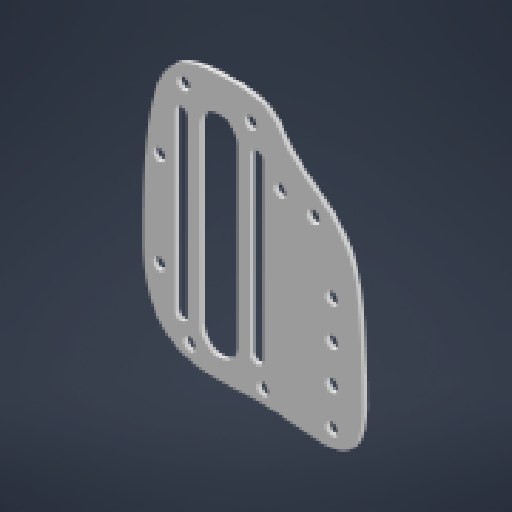
# Autodesk Inventor part: first-stage
Saved by Autodesk Inventor 2023.2 (Build 272271000, 271)
## iProperties
Created: 2023-03-31
Part Number: first-stage
Material: Generic
Document SubType Name: Modeling
Designer: eduar
Density: 1 g/cm^3
Appearance: Default
Author: eduar
Autodesk Inventor part; units mm, degrees
ref_plane "YZ Plane" through (0, 0, 0) normal (1, 0, 0) x (0, 1, 0)
ref_plane "XZ Plane" through (0, 0, 0) normal (0, 1, 0) x (-1, 0, 0)
ref_plane "XY Plane" through (0, 0, 0) normal (0, 0, 1) x (1, 0, 0)
sketch "Sketch1" plane through (0, 0, 0) normal (0, 0, 1) x (1, 0, 0)
  circle A0 centre (0, 139.7) radius 2.0955
  circle A1 centre (0, 127) radius 2.0955
  line L0 (-63.6282, 137.6045) -> (-63.6282, 111.7262) construction
  line L1 (-63.6282, 111.7262) -> (-38.1, 106.8497) construction
  line L2 (-38.1, 106.8497) -> (-23.3045, 114.3) construction
  line L3 (-23.3045, 114.3) -> (10.2927, 101.7972) construction
  line L4 (10.2927, 101.7972) -> (10.9951, 128.4781) construction
  line L5 (10.9951, 128.4781) -> (9.5904, 142.0848) construction
  line L6 (9.5904, 142.0848) -> (9.5904, 176.1435) construction
  line L7 (9.5904, 176.1435) -> (-18.114, 184.6297) construction
  line L8 (-18.114, 184.6297) -> (-19.6095, 190.621) construction
  line L9 (-19.6095, 190.621) -> (-43.1752, 188.9709) construction
  line L10 (-43.1752, 188.9709) -> (-63.6282, 188.9709) construction
  line L11 (-63.6282, 188.9709) -> (-63.6282, 149.1308) construction
  line L12 (-63.6282, 149.1308) -> (-63.6282, 137.6045) construction
  spline S0 degree 4 poles (-63.6282, 137.6045) (-63.6282, 111.7262) (-38.1, 106.8497) (-23.3045, 114.3) (10.2927, 101.7972) (10.9951, 128.4781) (9.5904, 142.0848) (9.5904, 176.1435) (-18.114, 184.6297) (-19.6095, 190.621) (-43.1752, 188.9709) (-63.6282, 188.9709) (-63.6282, 149.1308) (-63.6282, 137.6045) knots 0 0 0 0 0 1 2 3 4 5 6 7 8 9 10 10 10 10 10
  circle A2 centre (0, 114.3) radius 2.0955
  circle A3 centre (0, 152.4) radius 2.0955
  arc A4 (-31.75, 180.975) -> (-44.45, 180.975) centre (-38.1, 180.975) ccw
  line L13 (-44.45, 180.975) -> (-44.45, 122.555)
  line L14 (-31.75, 180.975) -> (-31.75, 122.555)
  arc A5 (-48.7045, 180.975) -> (-52.8955, 180.975) centre (-50.8, 180.975) ccw
  line L15 (-52.8955, 180.975) -> (-48.7045, 180.975) construction
  line L16 (-44.45, 180.975) -> (-31.75, 180.975) construction
  arc A6 (-23.3045, 180.975) -> (-27.4955, 180.975) centre (-25.4, 180.975) ccw
  line L17 (-23.3045, 180.975) -> (-27.4955, 180.975) construction
  line L18 (-23.3045, 180.975) -> (-23.3045, 122.555)
  line L19 (-27.4955, 180.975) -> (-27.4955, 122.555)
  line L20 (-48.7045, 180.975) -> (-48.7045, 122.555)
  line L21 (-52.8955, 180.975) -> (-52.8955, 122.555)
  arc A7 (-52.8955, 122.555) -> (-48.7045, 122.555) centre (-50.8, 122.555) ccw
  line L22 (-52.8955, 122.555) -> (-48.7045, 122.555) construction
  arc A8 (-44.45, 122.555) -> (-31.75, 122.555) centre (-38.1, 122.555) ccw
  line L23 (-44.45, 122.555) -> (-31.75, 122.555) construction
  arc A9 (-27.4955, 122.555) -> (-23.3045, 122.555) centre (-25.4, 122.555) ccw
  line L24 (-23.3045, 122.555) -> (-27.4955, 122.555) construction
  circle A10 centre (-6.35, 173.0375) radius 2.0955
  circle A11 centre (-48.0415, 115.1376) radius 2.0955
  circle A12 centre (-58.2851, 133.4575) radius 2.0955
  circle A13 centre (-58.2851, 165.3512) radius 2.0955
  circle A14 centre (-23.3045, 114.3) radius 2.0955
  circle A15 centre (-17.514, 175.133) radius 2.0955
  point P0 (0, 0)
  dimension "d17" = 4.191
  dimension "d18" = 4.191
  dimension "d19" = 4.191
  dimension "d20" = 4.191
  dimension "d23" = 6.35
  dimension "d24" = 12.7
  dimension "d25" = 2.0955
  dimension "d26" = 12.7
  dimension "d27" = 12.7
  dimension "d28" = 2.0955
  dimension "d29" = 58.42
  dimension "d30" = 4.191
  dimension "d31" = 4.191
  dimension "d32" = 4.191
  dimension "d33" = 4.191
  dimension "d36" = 4.191
  dimension "d37" = 4.191
  constraints: 24 end point, 16 centre point, 13 point on circle, 10 vertical, 6 horizontal, 5 parallel, 4 midpoint, 4 tangent, 3 coincident, 2 collinear, 1 perpendicular, 13 other
  measures "d17" diameter of A2
  measures "d18" diameter of A1
  measures "d19" diameter of A0
  measures "d20" diameter of A3
  measures "d23" radius of A4
  measures "d24" distance between parallel lines of L14 L13
  measures "d25" radius of A5
  measures "d26" distance of point (-50.8, 180.975) point (-38.1, 180.975)
  measures "d27" distance of point (-25.4, 180.975) A4.centre
  measures "d28" radius of A6
  measures "d29" distance of point (-38.1, 180.975) point (-38.1, 122.555)
  measures "d30" diameter of A10
  measures "d31" diameter of A11
  measures "d32" diameter of A12
  measures "d33" diameter of A13
  measures "d36" diameter of A14
  measures "d37" diameter of A15
extrude "Extrusion2" add sketch "Sketch1" along normal blind 1.524
equation "\"d18\" = d17"
equation "\"d19\" = d17"
equation "\"d20\" = d17"
equation "\"d24\" = 2 * d23"
body "Solid2"
